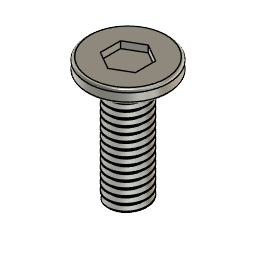
シノン_Tristan-bow_mk1_v42 (Autodesk Fusion 360 archive; units mm, degrees)
design "m3*8 _低頭ねじ"
Autodesk Fusion 360 part; units mm, degrees
sketch "スケッチ1" plane through (0, 0, 0) normal (0, 0, 1) x (1, 0, 0)
  circle A0 centre (0, 0) radius 3
  dimension "d1" = 6
  constraint coincident A0.centre origin
  measures "d1" diameter of A0
extrude "押し出し1" add sketch "スケッチ1" along normal blind 1
sketch "スケッチ2" plane through (0, 0, 0) normal (0, 0, -1) x (1, 0, 0)
  circle A0 centre (0, 0) radius 3
  circle A1 centre (0, 0) radius 1.5
  dimension "d4" = 3
  constraint coincident A0.centre A1.centre
  measures "d4" diameter of A1
extrude "押し出し2" add sketch "スケッチ2" along normal blind 8 contours A1
thread "ねじ1" "ISO Metric profile 3.0 M3x0.5 M3x0.5 6g" major diameter 2.927 minor diameter 2.3555 pitch 0.5 angle 60 modelled right hand crest width 0.0713 on face at (1.4981, 0.0748, -5.3333) crest through (1.4635, 0, 0.125)
fillet "フィレット1" radius 0.2 2 edges at (-2.797, -1.0848, 1) (-2.797, -1.0848, 0)
sketch "スケッチ3" plane through (0, 0, 1) normal (0, 0, 1) x (-1, 0, 0)
  circle A0 centre (0, 0) radius 2.8
  line L0 (0, -1.5) -> (1.299, -0.75)
  line L1 (1.299, -0.75) -> (1.299, 0.75)
  line L2 (1.299, 0.75) -> (0, 1.5)
  line L3 (0, 1.5) -> (-1.299, 0.75)
  line L4 (-1.299, 0.75) -> (-1.299, -0.75)
  line L5 (-1.299, -0.75) -> (0, -1.5)
  constraint coincident A0.centre origin
extrude "押し出し3" cut sketch "スケッチ3" against normal blind 0.5 contours L0 L1 L2 L3 L4 L5

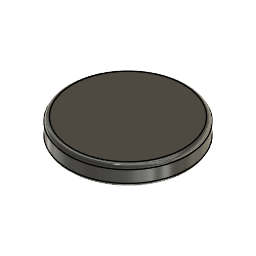
design "Φ6*1mm_ネオジム磁石"
Autodesk Fusion 360 part; units mm, degrees
sketch "スケッチ1" plane through (0, 0, 0) normal (0, 0, 1) x (1, 0, 0)
  circle A0 centre (0, 0) radius 3
  dimension "d1" = 6
  constraint coincident A0.centre origin
  measures "d1" diameter of A0
extrude "押し出し1" add sketch "スケッチ1" along normal blind 1
fillet "フィレット1" radius 0.2 2 edges at (-2.797, -1.0848, 1) (-2.797, -1.0848, 0)

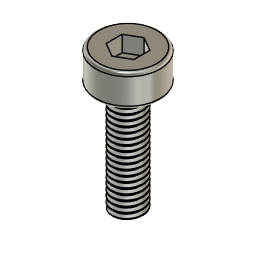
design "m3*10_六角ネジ"
Autodesk Fusion 360 part; units mm, degrees
sketch "スケッチ1" plane through (0, 0, 0) normal (0, 0, 1) x (1, 0, 0)
  circle A0 centre (0, 0) radius 3
  dimension "d1" = 6
  constraint coincident A0.centre origin
  measures "d1" diameter of A0
extrude "押し出し1" add sketch "スケッチ1" along normal blind 3
sketch "スケッチ2" plane through (0, 0, 0) normal (0, 0, -1) x (1, 0, 0)
  circle A0 centre (0, 0) radius 3
  circle A1 centre (0, 0) radius 1.5
  dimension "d4" = 3
  constraint coincident A0.centre A1.centre
  measures "d4" diameter of A1
extrude "押し出し2" add sketch "スケッチ2" along normal blind 10 contours A1
thread "ねじ1" "ISO Metric profile 3.0 M3x0.5 M3x0.5 6g" major diameter 2.927 minor diameter 2.3555 pitch 0.5 angle 60 modelled right hand crest width 0.0713 on face at (1.4981, 0.0748, -6.6667) crest through (1.4635, 0, 0.125)
fillet "フィレット1" radius 0.3 2 edges at (-2.797, -1.0848, 3) (-2.797, -1.0848, 0)
sketch "スケッチ3" plane through (0, 0, 3) normal (0, 0, 1) x (-1, 0, 0)
  circle A0 centre (0, 0) radius 2.7
  line L0 (0, -1.5) -> (1.299, -0.75)
  line L1 (1.299, -0.75) -> (1.299, 0.75)
  line L2 (1.299, 0.75) -> (0, 1.5)
  line L3 (0, 1.5) -> (-1.299, 0.75)
  line L4 (-1.299, 0.75) -> (-1.299, -0.75)
  line L5 (-1.299, -0.75) -> (0, -1.5)
  constraint coincident A0.centre origin
extrude "押し出し3" cut sketch "スケッチ3" against normal blind 1.5 contours L0 L1 L2 L3 L4 L5
